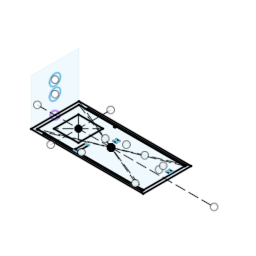
optical density standalone 4 v12 (Autodesk Fusion 360 design; units mm, degrees)
Autodesk Fusion 360 part; units mm, degrees
sketch "SketchBottom" plane through (0, 0, 0) normal (0, 0, 1) x (1, 0, 0)
  line L0 (-34.5, 13.6) -> (34.5, 13.6)
  line L1 (34.5, 13.6) -> (34.5, -13.6)
  line L2 (34.5, -13.6) -> (-34.5, -13.6)
  line L3 (-34.5, -13.6) -> (-34.5, 13.6)
  line L4 (-34.5, 13.6) -> (34.5, -13.6) construction
  line L5 (34.5, 13.6) -> (-34.5, -13.6) construction
  line L6 (-36.5, 15.6) -> (36.5, 15.6)
  line L7 (36.5, 15.6) -> (36.5, -15.6)
  line L8 (36.5, -15.6) -> (-36.5, -15.6)
  line L9 (-36.5, -15.6) -> (-36.5, 15.6)
  line L10 (-36.5, 15.6) -> (36.5, -15.6) construction
  line L11 (36.5, 15.6) -> (-36.5, -15.6) construction
  line L12 (34.5, 13.6) -> (-29.5, 13.6)
  line L13 (-29.5, 13.6) -> (-29.5, 14.6)
  line L14 (-29.5, 14.6) -> (34.5, 14.6)
  line L15 (34.5, 14.6) -> (34.5, 13.6)
  line L16 (0, 0) -> (67, 0) construction
  line L17 (34.5, -13.6) -> (-29.5, -13.6)
  line L18 (-29.5, -13.6) -> (-29.5, -14.6)
  line L19 (-29.5, -14.6) -> (34.5, -14.6)
  line L20 (34.5, -14.6) -> (34.5, -13.6)
  line L21 (0, 0) -> (-48, 0) construction
  line L22 (-10.7, 13.6) -> (-10, 13.6)
  line L23 (-10, 13.6) -> (-10, 12.6)
  line L24 (-10, 12.6) -> (-10.7, 12.6)
  line L25 (-10.7, 12.6) -> (-10.7, 13.6)
  line L26 (-10.7, -13.6) -> (-10, -13.6)
  line L27 (-10.7, -12.6) -> (-10.7, -13.6)
  line L28 (-10, -12.6) -> (-10.7, -12.6)
  line L29 (-10, -13.6) -> (-10, -12.6)
  circle A0 centre (28.0809, -12.3916) radius 1
  circle A1 centre (-6.9191, -12.3916) radius 1
  circle A2 centre (28.0809, 3.1084) radius 1
  circle A3 centre (-6.9191, 3.1084) radius 1
  line L30 (-10.7, -6) -> (-8.6, -6)
  line L31 (-8.6, -6) -> (-8.6, -13.6)
  line L32 (-8.6, -13.6) -> (-10.7, -13.6)
  line L33 (-10.7, -13.6) -> (-10.7, -6)
  line L34 (-2.9377, 6.4) -> (-0.9377, 6.4)
  line L35 (-0.9377, 6.4) -> (-0.9377, 4.4)
  line L36 (-0.9377, 4.4) -> (-2.9377, 4.4)
  line L37 (-2.9377, 4.4) -> (-2.9377, 6.4)
  line L38 (33.5623, 4.4) -> (31.5623, 4.4)
  line L39 (31.5623, 4.4) -> (31.5623, 6.4)
  line L40 (33.5623, 6.4) -> (33.5623, 4.4)
  line L41 (31.5623, 6.4) -> (33.5623, 6.4)
  line L42 (-21.25, 21) -> (-21.25, -18) construction
  line L43 (-29.25, 8) -> (-13.25, 8)
  line L44 (-13.25, 8) -> (-13.25, -8)
  line L45 (-13.25, -8) -> (-29.25, -8)
  line L46 (-29.25, -8) -> (-29.25, 8)
  line L47 (-29.25, 8) -> (-13.25, -8) construction
  line L48 (-13.25, 8) -> (-29.25, -8) construction
  circle A4 centre (3.3763, 6.5863) radius 1
  circle A5 centre (15.3263, 6.5863) radius 1
  circle A6 centre (27.2763, 6.5863) radius 1
  point P0 (-21.25, 0)
  dimension "d8" = 69
  dimension "d9" = 27.2
  dimension "d10" = 73
  dimension "d12" = 31.2
  dimension "d13" = 64
  dimension "d14" = 1
  dimension "d15" = 0.7
  dimension "d16" = 1
  dimension "d19" = 2
  dimension "d22" = -35
  dimension "d23" = 15.5
  dimension "d25" = 7.6
  dimension "d26" = 43.1
  dimension "d27" = 2
  dimension "d28" = 2
  dimension "d29" = 18
  dimension "d32" = 34.5
  dimension "d33" = 0
  dimension "d74" = 13.25
  dimension "d75" = 44.5
  dimension "d76" = 16
  dimension "d77" = 16
  dimension "d107" = 2
  dimension "d110" = 23.9
  dimension "d111" = 0
  constraint horizontal L0
  constraint perpendicular L0 L1
  constraint parallel L0 L2
  constraint parallel L1 L3
  constraint coincident L4 L16.start
  constraint coincident L5 L16.start
  constraint coincident L16.start L21.start
  constraint horizontal L6
  constraint perpendicular L6 L7
  constraint parallel L6 L8
  constraint parallel L7 L9
  constraint coincident L10 L16.start
  constraint coincident L11 L16.start
  constraint horizontal L12
  constraint vertical L13
  constraint horizontal L14
  constraint vertical L15
  constraint perpendicular L7 L16
  constraint symmetric L0.end L16 L1.end
  constraint symmetric L12.end L16 L17.end
  constraint symmetric L13.end L16 L18.end
  constraint symmetric L14.end L16 L19.end
  constraint horizontal L21
  constraint horizontal L22
  constraint vertical L23
  constraint horizontal L24
  constraint vertical L25
  constraint coincident L0 L22.start
  constraint symmetric L21 L22.start L26.start
  constraint symmetric L21 L22.end L26.end
  constraint symmetric L21 L23.end L28.start
  constraint symmetric L21 L24.end L27.start
  constraint horizontal L30
  constraint vertical L31
  constraint horizontal L32
  constraint vertical L33
  constraint horizontal L34
  constraint vertical L35
  constraint horizontal L36
  constraint vertical L37
  constraint perpendicular L8 L42
  constraint horizontal L43
  constraint perpendicular L43 L44
  constraint parallel L43 L45
  constraint parallel L44 L46
  constraint coincident L47 P0
  constraint coincident L48 P0
  constraint coincident L21 P0
  constraint coincident L42 P0
  constraint collinear L25 L33
  measures "d8" distance of L1.end L2.end
  measures "d9" distance of L0.start L2.end
  measures "d10" distance of L7.end L8.end
  measures "d12" distance of L6.start L8.end
  measures "d13" distance of L0.end L12.end
  measures "d14" distance of L0.end L14.end
  measures "d15" distance of L22.start L22.end
  measures "d16" distance of L22.start L24.end
  measures "d19" diameter of A0
  measures "d25" distance of L30.start L26.start
  measures "d26" distance of L1 L31.end
  measures "d27" distance of L34.start L34.end
  measures "d28" distance of L34.start L36.end
  measures "d29" distance of L2 L35.end
  measures "d74" distance of L3 L42
  measures "d75" distance of L1 L23
  measures "d76" distance of L44.end L45.end
  measures "d77" distance of L43.end L44.end
  measures "d107" diameter of A4
extrude "Extrude1" add sketch "SketchBottom" along normal blind 10 contours L2 L17 L26 L27 L28 L29 L32 L33 | L2 L17 L28 L29 L30 L31 L32 L33 makes body 1
extrude "Extrude2" add sketch "SketchBottom" along normal blind 3.5 separate body contours A0 | A1 | A2 | A3 makes body 2 at (-5.9241, -12.4911, 2.3333) makes body 3 at (29.0759, -12.4911, 2.3333) makes body 4 at (-5.9241, 3.0089, 2.3333) makes body 5 at (29.0759, 3.0089, 2.3333)
extrude "Extrude3" add sketch "SketchBottom" along normal blind 7 separate body contours L34 L35 L36 L37 | L38 L39 L40 L41 makes body 6 at (-0.9377, 5.7333, 2.3333) makes body 7 at (33.5623, 5.7333, 2.3333)
chamfer "Chamfer1" distance 2 angle 45 1 edges at (-8.6, -9.8, 10) on bodies 1
fillet "Fillet2" radius 0.7 1 edges at (-10.7, -9.8, 10) on bodies 1
extrude "Extrude4" add sketch "SketchBottom" along normal blind 2 contours L0 L1 L2 L3 L12 L17 L23 L24 L25 L27 L30 L31 L33 | L43 L44 L45 L46 | A4 | A5 | A6 bodies 1 2 3 4 5 6 7
extrude "Extrude5" add sketch "SketchBottom" along normal blind 22 contours L0 L12 L22 L23 L24 L25 bodies 1
extrude "Extrude6" add sketch "SketchBottom" along normal blind 30 contours L0 L12 L13 L14 L15 L22 | L2 L17 L18 L19 L20 L26 L32 | L6 L7 L8 L9 bodies 1
sketch "USBSketch" plane through (36.5, 0, 0) normal (1, 0, 0) x (0, 1, 0)
  line L0 (-15.6, 0) -> (15.6, 0)
  line L1 (15.6, 0) -> (15.6, 30)
  line L2 (15.6, 30) -> (-15.6, 30)
  line L3 (-15.6, 30) -> (-15.6, 0)
  line L4 (0, 0) -> (0, 33) construction
  line L5 (15.6, 0) -> (-15.6, 0)
  line L6 (-4.27, 1.2334) -> (-4.27, 42.2334) construction
  line L7 (-7.67, 8.1) -> (-4.27, 8.1)
  line L8 (-0.87, 7.4) -> (-0.87, 6.1)
  line L9 (-0.87, 6.1) -> (-7.67, 6.1)
  line L10 (-7.67, 6.1) -> (-7.67, 7.4)
  line L11 (-7.67, 8.1) -> (-0.87, 6.1) construction
  line L12 (-0.87, 8.1) -> (-7.67, 6.1) construction
  line L13 (-8.27, 8.1) -> (-8.27, 9.8)
  line L14 (-7.97, 10.1) -> (-0.57, 10.1)
  line L15 (-0.27, 9.8) -> (-0.27, 8.1)
  line L16 (-0.27, 8.1) -> (-8.27, 10.1) construction
  line L17 (-8.27, 8.1) -> (-0.27, 10.1) construction
  line L18 (-0.27, 8.1) -> (-0.17, 8.1)
  line L19 (-8.37, 8.1) -> (-8.27, 8.1)
  arc A0 (-7.67, 7.4) -> (-8.37, 8.1) centre (-8.37, 7.4) ccw
  arc A1 (-0.17, 8.1) -> (-0.87, 7.4) centre (-0.17, 7.4) ccw
  arc A2 (-7.97, 10.1) -> (-8.27, 9.8) centre (-7.97, 9.8) ccw
  arc A3 (-0.27, 9.8) -> (-0.57, 10.1) centre (-0.57, 9.8) ccw
  point P0 (-4.27, 7.1)
  point P1 (-4.27, 9.1)
  dimension "d56" = 11.33
  dimension "d57" = 6.1
  dimension "d58" = 6.8
  dimension "d59" = 8
  dimension "d60" = 2
  dimension "d61" = 2
  dimension "d62" = 0.7
  dimension "d63" = 0.7
  dimension "d64" = 0.3
  dimension "d65" = 0.3
  constraint coincident L4.start origin
  constraint perpendicular L0 L4
  constraint horizontal L7
  constraint perpendicular L7 L8
  constraint parallel L7 L9
  constraint parallel L8 L10
  constraint coincident L11 P0
  constraint coincident L12 P0
  constraint coincident L6 P0
  constraint horizontal L18
  constraint perpendicular L13 L18
  constraint parallel L14 L18
  constraint parallel L13 L15
  constraint coincident L16 P1
  constraint coincident L17 P1
  constraint coincident L6 P1
  constraint collinear L7 L18
  constraint coincident L6 L7.end
  constraint collinear L18 L19
  constraint coincident L7.start L10
  constraint tangent L10 A0
  constraint tangent L19 A0
  constraint coincident L12.start L18
  constraint coincident L12.start L8
  constraint tangent L18 A1
  constraint tangent L8 A1
  constraint coincident L16.end L13
  constraint coincident L16.end L14
  constraint tangent L13 A2
  constraint tangent L14 A2
  constraint coincident L17.end L14
  constraint coincident L17.end L15
  constraint tangent L14 A3
  constraint tangent L15 A3
  measures "d56" distance of L3 L6
  measures "d57" distance of L5 L9
  measures "d58" distance of L8.end L9.end
  measures "d59" distance of L16.end L17.end
  measures "d60" distance of L12.start L8.end
  measures "d61" distance of L15.end L17.end
  measures "d62" radius of A0
  measures "d63" radius of A1
  measures "d64" radius of A2
  measures "d65" radius of A3
extrude "Extrude7" cut sketch "USBSketch" against normal blind 2 contours L8 L9 L10 L13 L14 L15 L18 L19 A0 A1 A2 A3 bodies 1
extrude "Extrude8" cut sketch "SketchBottom" along normal blind 3 from surface at 26 contours L0 L12 L13 L14 L15 L22 | L2 L17 L18 L19 L20 L26 L32 bodies 1
sketch "SketchVentilationHoles" plane through (-36.5, 0, 0) normal (-1, 0, 0) x (0, -1, 0)
  line L0 (-15.6, 0) -> (15.6, 0)
  line L1 (15.6, 0) -> (15.6, 30)
  line L2 (15.6, 30) -> (-15.6, 30)
  line L3 (-15.6, 30) -> (-15.6, 0)
  circle A0 centre (0, 19.9799) radius 3.5
  circle A1 centre (0, 11.7998) radius 3.5
  dimension "d71" = 7
  dimension "d104" = 7
  constraint vertical A0.centre A1.centre
  constraint vertical A1.centre origin
  measures "d71" diameter of A0
  measures "d104" diameter of A1
extrude "Extrude9" cut sketch "SketchVentilationHoles" against normal blind 2 contours A0 | A1 bodies 1
extrude "Extrude10" cut sketch "SketchBottom" along normal blind 2 contours L43 L44 L45 L46 bodies 1
sketch "Sketch1" plane through (0, 0, 0) normal (0, 0, 1) x (1, 0, 0) in component "lid"
  line L0 (-36.5, 15.6) -> (36.5, 15.6)
  line L1 (36.5, 15.6) -> (36.5, -15.6)
  line L2 (36.5, -15.6) -> (-36.5, -15.6)
  line L3 (-36.5, -15.6) -> (-36.5, 15.6)
  line L4 (-36.5, 15.6) -> (36.5, -15.6) construction
  line L5 (36.5, 15.6) -> (-36.5, -15.6) construction
  line L6 (-23.8635, -13.9902) -> (-21.8635, -13.9902)
  line L7 (-21.8635, -13.9902) -> (-21.8635, -11.9902)
  line L8 (-21.8635, -11.9902) -> (-23.8635, -11.9902)
  line L9 (-23.8635, -11.9902) -> (-23.8635, -13.9902)
  line L10 (31.5365, -11.9902) -> (31.5365, -13.9902)
  line L11 (31.5365, -13.9902) -> (33.5365, -13.9902)
  line L12 (33.5365, -13.9902) -> (33.5365, -11.9902)
  line L13 (33.5365, -11.9902) -> (31.5365, -11.9902)
  line L14 (-23.8635, 14.0098) -> (-23.8635, 12.0098)
  line L15 (-23.8635, 12.0098) -> (-21.8635, 12.0098)
  line L16 (-21.8635, 12.0098) -> (-21.8635, 14.0098)
  line L17 (-21.8635, 14.0098) -> (-23.8635, 14.0098)
  line L18 (31.5365, 14.0098) -> (31.5365, 12.0098)
  line L19 (31.5365, 12.0098) -> (33.5365, 12.0098)
  line L20 (33.5365, 12.0098) -> (33.5365, 14.0098)
  line L21 (33.5365, 14.0098) -> (31.5365, 14.0098)
  line L22 (-21.25, 11) -> (-21.25, -21) construction
  line L23 (-36.5, -15.6) -> (-36.5, 15.6)
  line L24 (-13.5, -7.75) -> (-29, -7.75)
  line L25 (-29, -7.75) -> (-29, 7.75)
  line L26 (-29, 7.75) -> (-13.5, 7.75)
  line L27 (-13.5, 7.75) -> (-13.5, -7.75)
  line L28 (-13.5, -7.75) -> (-29, 7.75) construction
  line L29 (-29, -7.75) -> (-13.5, 7.75) construction
  line L30 (-23.8635, 13.5984) -> (-21.8635, 13.5984)
  line L31 (31.5365, 13.5984) -> (33.5365, 13.5984)
  line L32 (31.5365, -13.6218) -> (33.5365, -13.6218)
  line L33 (-23.8635, -13.5943) -> (-21.8635, -13.5943)
  line L34 (34.3, 0.867) -> (32.3, 0.867)
  line L35 (32.3, 0.867) -> (32.3, -1.133)
  line L36 (32.3, -1.133) -> (34.3, -1.133)
  line L37 (34.3, -1.133) -> (34.3, 0.867)
  line L38 (0, 18) -> (0, -23) construction
  line L39 (-32.3, -1.133) -> (-34.3, -1.133)
  line L40 (-34.3, -1.133) -> (-34.3, 0.867)
  line L41 (-32.3, 0.867) -> (-32.3, -1.133)
  line L42 (-34.3, 0.867) -> (-32.3, 0.867)
  point P0 (-21.25, 0)
  dimension "d80" = 73
  dimension "d81" = 31.2
  dimension "d82" = 2
  dimension "d83" = 2
  dimension "d86" = 55.4
  dimension "d87" = 26
  dimension "d90" = 15.25
  dimension "d91" = 15.5
  dimension "d92" = 15.5
  dimension "d124" = 2
  dimension "d125" = 2
  dimension "d126" = 2.2
  constraint horizontal L0
  constraint perpendicular L0 L1
  constraint parallel L0 L2
  constraint parallel L1 L3
  constraint coincident L4 origin
  constraint coincident L5 origin
  constraint horizontal L6
  constraint vertical L7
  constraint horizontal L8
  constraint vertical L9
  constraint perpendicular L2 L22
  constraint horizontal L24
  constraint perpendicular L24 L25
  constraint parallel L24 L26
  constraint parallel L25 L27
  constraint coincident L28 P0
  constraint coincident L29 P0
  constraint coincident L22 P0
  constraint coincident L14 L30.start
  constraint coincident L16 L30.end
  constraint perpendicular L16 L30
  constraint coincident L18 L31.start
  constraint coincident L20 L31.end
  constraint perpendicular L20 L31
  constraint coincident L10 L32.start
  constraint coincident L12 L32.end
  constraint perpendicular L12 L32
  constraint coincident L9 L33.start
  constraint coincident L7 L33.end
  constraint perpendicular L7 L33
  constraint horizontal origin P0
  constraint horizontal L34
  constraint vertical L35
  constraint horizontal L36
  constraint vertical L37
  constraint perpendicular L2 L38
  constraint symmetric L34.start L38 L40.end
  constraint symmetric L34.end L38 L41.start
  constraint symmetric L35.end L38 L39.start
  constraint symmetric L36.end L38 L39.end
  measures "d80" distance of L0.start L0.end
  measures "d81" distance of L0.start L2.end
  measures "d82" distance of L6.start L6.end
  measures "d83" distance of L6.start L8.end
  measures "d90" distance of L22 L23
  measures "d91" distance of L25.end L26.end
  measures "d92" distance of L24.end L25.end
  measures "d124" distance of L34.start L34.end
  measures "d125" distance of L34.start L36.end
  measures "d126" distance of L1 L37
extrude "Extrude2'" add sketch "Sketch1" along normal blind 2 separate body contours L0 L1 L2 L3 L23 | L34 L35 L36 L37 | L39 L40 L41 L42 makes body 8 in component "lid"
extrude "Extrude3'" add sketch "Sketch1" along normal blind 4.5 contours L6 L7 L9 L33 | L7 L8 L9 L33 | L10 L12 L13 L32 | L10 L11 L12 L32 | L14 L16 L17 L30 | L14 L15 L16 L30 | L18 L20 L21 L31 | L18 L19 L20 L31 bodies 8 in component "lid"
extrude "Extrude4'" cut sketch "Sketch1" along normal blind 1.5 from surface at 2 contours L6 L7 L9 L33 | L10 L11 L12 L32 | L14 L16 L17 L30 | L18 L20 L21 L31 bodies 8 in component "lid"
extrude "Extrude13" cut sketch "SketchBottom" along normal blind 2 contours A4 | A5 | A6 bodies 1
fillet "Fillet1" radius 1 4 edges at (-22.8635, -13.9902, 4.5) (32.5365, -13.9902, 4.5) (32.5365, 14.0098, 4.5) (-22.8635, 14.0098, 4.5) on bodies 8 in component "lid"
fillet "Fillet2'" radius 0.3 4 edges at (32.5365, -13.9902, 3.5) (-22.8635, 14.0098, 3.5) (-22.8635, -13.9902, 3.5) (32.5365, 14.0098, 3.5) on bodies 8 in component "lid"
fillet "Fillet1'" radius 1 1 edges at (-10.7, 13.1, 22) on bodies 1
sketch "text" plane through (0, 15.6, 0) normal (0, 1, 0) x (-1, 0, 0)
  line L0 (-36.5, 0) -> (36.5, 0)
  line L1 (36.5, 0) -> (36.5, 30)
  line L2 (36.5, 30) -> (-36.5, 30)
  line L3 (-36.5, 30) -> (-36.5, 0)
  line L4 (-33.6173, 12) -> (34.4083, 12) construction
  line L5 (34.4083, 12) -> (34.4083, 25) construction
  line L6 (34.4083, 25) -> (-33.6173, 25) construction
  line L7 (-33.6173, 25) -> (-33.6173, 12) construction
  dimension "d121" = 7
  text T0 "Optical Density" font "Arial" height 7 align left top in box 68.0257 x 13 at (-33.6173, 12) x (1, 0) y (0, 1) spacing 1 kerned
extrude "Extrude14" add sketch "text" along normal blind 0.3 text T0 bodies 1
extrude "Extrude5'" add sketch "Sketch1" along normal blind 5 contours L34 L35 L36 L37 | L39 L40 L41 L42 bodies 8 in component "lid"
component "lid" placed x (1, 0, 0) y (0, 1, 0) z (0, 0, 1) at (0, 0, 0)
equation "internalNanoHousigLen = 44.5 mm"
equation "internalWidth = 31.2 mm - 4 mm"
equation "internalInsertLen = 24.5 mm"
equation "NanoStoppeInternalLen = 43.1 mm"
equation "height = 30 mm"
equation "d8 = internalNanoHousigLen + internalInsertLen"
equation "d9 = internalWidth"
equation "d10 = internalNanoHousigLen + internalInsertLen + 2 * wallThickness"
equation "wallThickness = 2 mm"
equation "d12 = internalWidth + 2 * wallThickness"
equation "d13 = internalNanoHousigLen + internalInsertLen - 5 mm"
equation "compartmentSeparatorHeight = height - 8 mm"
equation "d19 = wallThickness"
equation "d26 = NanoStoppeInternalLen"
equation "d27 = wallThickness"
equation "d28 = wallThickness"
equation "d41 = wallThickness"
equation "d43 = compartmentSeparatorHeight"
equation "d45 = height"
equation "UsbWidth = 5.9 mm"
equation "UsbTopRectangleWidth = 8 mm"
equation "UsbBottomRectangleWidth = 6.8 mm"
equation "UsbTopRectangleHeight = 2 mm"
equation "UsbBottomRectangleHeight = 2 mm"
equation "UsbVerticalMedian = wallThickness + 7.33 mm"
equation "d56 = UsbVerticalMedian + wallThickness"
equation "d57 = 4.1 mm + wallThickness"
equation "d58 = UsbBottomRectangleWidth"
equation "d59 = UsbTopRectangleWidth"
equation "d60 = UsbBottomRectangleHeight"
equation "d61 = UsbTopRectangleHeight"
equation "d66 = -wallThickness"
equation "d68 = height - 4 mm"
equation "d72 = -wallThickness"
equation "d74 = ( internalNanoHousigLen + internalInsertLen + 2 * wallThickness - internalNanoHousigLen - wallThickness ) / 2"
equation "d75 = internalNanoHousigLen"
equation "d78 = wallThickness"
equation "d80 = internalInsertLen + internalNanoHousigLen + 2 * wallThickness"
equation "d81 = internalWidth + 2 * wallThickness"
equation "d82 = wallThickness"
equation "d83 = wallThickness"
equation "d90 = 13.25 mm + wallThickness"
equation "d93 = wallThickness"
equation "d95 = wallThickness + 2.5 mm"
equation "d99 = wallThickness"
equation "d107 = wallThickness"
equation "d116 = wallThickness"
equation "d124 = wallThickness"
equation "d125 = wallThickness"
